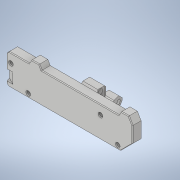
# Autodesk Inventor part: MINI-y-plate-rear
Saved by Autodesk Inventor 2021 (Build 250183000, 183)
## iProperties
Company: Prusa Development a.s.
RuleStatus: InUse
Created: 2019-07-31
Material: Všeobecné
Document SubType Name: Modeling
Density: 1 g/cm^3
Appearance: Výchozí
Project: ORIGINAL PRUSA MINI
Authority: Ing. Robert Turinský
Author: Ing. Robert Turinský
Title: MINI-y-plate-rear
Revision Number: R4
Autodesk Inventor part; units mm, degrees
(part 1 of 2)
ref_plane "XY Plane" through (0, 0, 0) normal (0, 0, 1) x (1, 0, 0)
sketch "Náčrt1" plane through (0, 0, 0) normal (0, 0, 1) x (1, 0, 0)
  line L0 (0, -49.6) -> (0, 14.1) projected
  line L1 (-71.6, 0) -> (163.6, 0) projected
  arc A0 (0.375, -4.0577) -> (-0.375, -4.0577) centre (0, 0) ccw
  arc A1 (120.375, -4.0577) -> (119.625, -4.0577) centre (120, 0) ccw
  line L2 (5, 5) -> (-5, 5)
  line L3 (-5, 5) -> (-8.1754, -0.5)
  line L4 (-8.1754, -0.5) -> (-35.5, -0.5)
  line L5 (-35.5, -0.5) -> (-38, -3)
  line L6 (-38, -3) -> (-38, -38)
  line L7 (-38, -38) -> (-35.5, -40.5)
  line L8 (-35.5, -40.5) -> (114, -40.5)
  line L9 (114, -40.5) -> (130, -24.5)
  line L10 (130, -24.5) -> (130, -3.6603)
  line L11 (130, -3.6603) -> (125, 5)
  line L12 (125, 5) -> (115, 5)
  line L13 (115, 5) -> (111.8246, -0.5)
  line L14 (111.8246, -0.5) -> (8.1754, -0.5)
  line L15 (8.1754, -0.5) -> (5, 5)
  circle A2 centre (87.45, -12.35) radius 2.65
  circle A3 centre (110.7, -35.6) radius 2.65
  circle A4 centre (-32.55, -12.35) radius 2.65
  circle A5 centre (-9.3, -35.6) radius 2.65
  line L16 (119.625, -4.0577) -> (119.625, -12)
  line L17 (119.625, -12) -> (120.375, -12)
  line L18 (120.375, -12) -> (120.375, -4.0577)
  line L19 (-0.375, -4.0577) -> (-0.375, -12)
  line L20 (-0.375, -12) -> (0.375, -12)
  line L21 (0.375, -12) -> (0.375, -4.0577)
  point P0 (120, 5)
  point P1 (0, 5)
  dimension "d0" = 8.15
  dimension "d1" = 120
  dimension "d2" = 0.5
  dimension "d3" = 5.5
  dimension "d4" = 10
  dimension "d5" = 60
  dimension "d6" = 2.5
  dimension "d7" = 2.5
  dimension "d8" = 38
  dimension "d9" = 40.5
  dimension "d10" = 168
  dimension "d11" = 16
  dimension "d12" = 5.3
  dimension "d13" = 5.45
  dimension "d14" = 28.15
  dimension "d15" = 23.25
  dimension "d16" = 23.25
  dimension "d17" = 23.25
  dimension "d18" = 120
  dimension "d25" = 0.75
  dimension "d26" = 12
  constraints: 40 end point, 7 equal length, 6 centre point, 6 parallel, 5 point on line, 4 equal radius, 4 point on circle, 3 perpendicular, 2 horizontal alignment, 2 midpoint, 2 vertical, 2 vertical alignment, 1 coincident, 1 collinear, 1 horizontal
  measures "d0" diameter of A0
  measures "d1" distance of A0.centre A1.centre
  measures "d2" distance between parallel lines of L1 L4
  measures "d3" distance between parallel lines of L4 L2
  measures "d4" distance of L2.start L2.end
  measures "d5" angle of L2 L3
  measures "d6" horizontal distance of L4.end L5.end
  measures "d7" horizontal distance of L4.end L5.end
  measures "d8" distance between parallel lines of L6 L0
  measures "d9" distance between parallel lines of L8 L1
  measures "d10" distance between parallel lines of L6 L10
  measures "d11" horizontal distance of L8.end L9.end
  measures "d12" diameter of A2
  measures "d13" distance from line of L6 A4.centre
  measures "d14" distance from line of L8 A4.centre
  measures "d15" horizontal distance of A5.centre A4.centre
  measures "d16" horizontal distance of A4.centre A5.centre
  measures "d17" horizontal distance of A2.centre A3.centre
  measures "d18" distance of A4.centre A2.centre
  measures "d25" distance between parallel lines of L16 L18
  measures "d26" distance between parallel lines of L17 L1
extrude "Vysunutí1" add sketch "Náčrt1" along normal blind 11.95 contours L8 L7 L6 L5 L4 L3 L1 A0 L19 L20 L0 | L0 L20 L21 A0 L1 L15 L14 L13 A1 L16 L17 L18 L11 L10 L9 L8 | A0 L1 L3 L2 L0 | L0 L2 L15 L1 A0 | L1 A1 L13 L12 L11
extrude "Vysunutí2" [suppressed]
sketch "Náčrt2" plane through (0, 0, 11.95) normal (0, 0, 1) x (1, 0, 0)
  arc A0 (120.375, -4.0577) -> (119.625, -4.0577) centre (120, 0) ccw projected
  arc A1 (0.375, -4.0577) -> (-0.375, -4.0577) centre (0, 0) ccw projected
  circle A2 centre (-9.3, -35.6) radius 2.65 projected
  circle A3 centre (-32.55, -12.35) radius 2.65 projected
  circle A4 centre (110.7, -35.6) radius 2.65 projected
  circle A5 centre (87.45, -12.35) radius 2.65 projected
  line L0 (5, 5) -> (-5, 5) projected
  line L1 (-5, 5) -> (-8.1754, -0.5) projected
  line L2 (-8.1754, -0.5) -> (-35.5, -0.5) projected
  line L3 (-35.5, -0.5) -> (-38, -3) projected
  line L4 (-38, -3) -> (-38, -38) projected
  line L5 (-38, -38) -> (-35.5, -40.5) projected
  line L6 (-35.5, -40.5) -> (114, -40.5) projected
  line L7 (114, -40.5) -> (130, -24.5) projected
  line L8 (130, -24.5) -> (130, -3.6603) projected
  line L9 (130, -3.6603) -> (125, 5) projected
  line L10 (125, 5) -> (115, 5) projected
  line L11 (115, 5) -> (111.8246, -0.5) projected
  line L12 (111.8246, -0.5) -> (8.1754, -0.5) projected
  line L13 (8.1754, -0.5) -> (5, 5) projected
  line L14 (120.375, -4.0577) -> (120.375, -12) projected
  line L15 (120.375, -12) -> (119.625, -12) projected
  line L16 (119.625, -12) -> (119.625, -4.0577) projected
  line L17 (0.375, -4.0577) -> (0.375, -12) projected
  line L18 (0.375, -12) -> (-0.375, -12) projected
  line L19 (-0.375, -12) -> (-0.375, -4.0577) projected
extrude "Vysunutí3" add sketch "Náčrt2" against normal blind 2 contours L14 L15 L16 A0 | L17 L18 L19 A1
ref_plane "Pracovní rovina1" through (50, 0, 0) normal (1, 0, 0) x (0, 1, 0)
sketch "Náčrt3" plane through (50, 0, 0) normal (1, 0, 0) x (0, 1, 0)
  line L0 (-0.5, 0) -> (-0.5, 11.95) projected
  line L1 (-48.9, 0) -> (9.9, 0) projected
  line L2 (0, -53.99) -> (0, 22.94) projected
  circle A0 centre (-18, -21) radius 11.25
  line L3 (-0.5, 0) -> (1.5, -2)
  line L4 (1.5, -2) -> (1.5, -11)
  line L5 (1.5, -11) -> (-0.5, -13)
  line L6 (-0.5, -13) -> (-10.0904, -13)
  line L7 (-26.5, -28.3697) -> (-26.5, -37)
  line L8 (-26.5, -37) -> (-32.5, -43)
  line L9 (-32.5, -43) -> (-36, -43)
  line L10 (-36, -43) -> (-39, -40)
  line L11 (-39, -40) -> (-40.5, -27)
  line L12 (-40.5, -27) -> (-40.5, 0)
  line L13 (-0.5, 0) -> (-0.5, 11.95) projected
  line L14 (-40.5, 0) -> (-0.5, 0)
  line L15 (-40.5, 0) -> (-40.5, 11.95) projected
  circle A1 centre (-2.5, -5.5) radius 1.7
  circle A2 centre (-33.5, -5.5) radius 1.7
  circle A3 centre (-33.5, -36.5) radius 1.7
  point P0 (0, 0)
  dimension "d28" = 22.5
  dimension "d29" = 21
  dimension "d30" = 18
  dimension "d31" = 8
  dimension "d32" = 19.5
  dimension "d33" = 45
  dimension "d34" = 8.5
  dimension "d35" = 6
  dimension "d36" = 22
  dimension "d37" = 3
  dimension "d38" = 13
  dimension "d39" = 1.5
  dimension "d40" = 3.4
  dimension "d41" = 31
  dimension "d42" = 31
  dimension "d43" = 15.5
  dimension "d44" = 15.5
  constraints: 22 end point, 5 perpendicular, 4 centre point, 3 vertical, 2 equal radius, 2 horizontal, 2 point on circle, 2 point on line, 1 horizontal alignment, 1 vertical alignment
  measures "d28" diameter of A0
  measures "d29" distance from line of L1 A0.centre
  measures "d30" distance from line of L2 A0.centre
  measures "d31" distance from line of A0.centre L6
  measures "d32" distance from line of A0.centre L4
  measures "d33" angle of L1 L3
  measures "d34" distance from line of L7 A0.centre
  measures "d35" horizontal distance of L7.end L8.end
  measures "d36" distance from line of A0.centre L9
  measures "d37" horizontal distance of L9.end L10.end
  measures "d38" vertical distance of L10.end L11.end
  measures "d39" horizontal distance of L10.end L11.end
  measures "d40" diameter of A1
  measures "d41" distance of A2.centre A1.centre
  measures "d42" distance of A3.centre A2.centre
  measures "d43" horizontal distance of A0.centre A2.centre
  measures "d44" horizontal distance of A0.centre A2.centre
extrude "Vysunutí4" add sketch "Náčrt3" along normal blind 20 contours L1 L3 L2 L5 L6 A0 L7 L8 L9 L10 L11 L12 | L3 L4 L5 L2
sketch "Náčrt4" plane through (0, 0, 0) normal (0, 1, 0) x (-1, 0, 0)
  line L0 (35.5, 0) -> (-50, 0) projected
  line L1 (-50, 0) -> (-50, -27) projected
  line L2 (-50, -27) -> (-70, -27) projected
  line L3 (-70, 0) -> (-70, -27) projected
  line L4 (-70, 0) -> (-114, 0) projected
  line L5 (-114, 0) -> (-114, 11.95) projected
  line L6 (35.5, 11.95) -> (-114, 11.95) projected
  line L7 (35.5, 0) -> (35.5, 11.95) projected
  line L8 (-50, -27) -> (-50, -40) projected
  line L9 (-50, -40) -> (-70, -40) projected
  line L10 (-70, -27) -> (-70, -40) projected
  line L11 (-50, -27) -> (-70, -27) projected
  line L12 (-50, -40) -> (-50, -43) projected
  line L13 (-50, -43) -> (-70, -43) projected
  line L14 (-70, -40) -> (-70, -43) projected
  line L15 (-50, -40) -> (-70, -40) projected
  line L16 (-61.5, -43) -> (-70, -43)
  line L17 (-70, -43) -> (-70, -11.2776)
  line L18 (-70, -11) -> (-70, -2) projected
  line L19 (-70, -11.2776) -> (-61.5, -43)
  point P0 (0, 0)
  dimension "d47" = 15
  dimension "d48" = 8.5
  constraints: 6 end point, 2 point on line, 1 horizontal
  measures "d47" angle of L14 L19
  measures "d48" horizontal distance of L17.end L16.start
extrude "Vysunutí5" cut sketch "Náčrt4" along normal through all both and the other way through all contours L19 L9 L10 L2 | L2 L3 L19 | L19 L13 L14 L9
sketch "Náčrt5" plane through (70, 0, 0) normal (1, 0, 0) x (0, 0, -1)
  point P0 (0, 0)
  point P1 (5.5, -2.5)
  point P2 (5.5, -33.5)
  point P3 (36.5, -33.5)
hole "Díra1" at (70, -2.5, -5.5) at (70, -33.5, -5.5) at (70, -33.5, -36.5) direction (-1, 0, 0) diameter 3.4 end through all counterbore diameter 6 counterbore depth 11
ref_plane "Pracovní rovina2" through (0, -23.975, 0) normal (0, 1, 0) x (-1, 0, 0)
sketch "Náčrt6" plane through (0, -23.975, 0) normal (0, 1, 0) x (-1, 0, 0)
  line L0 (-111.8246, 0) -> (-70, 0) projected
  line L1 (-115, 0) -> (-111.8246, 0) projected
  line L2 (-125, 0) -> (-115, 0) projected
  line L3 (-130, 0) -> (-125, 0) projected
  line L4 (-114, 0) -> (-130, 0) projected
  line L5 (-70, 0) -> (-114, 0) projected
  line L6 (-120.375, 0) -> (-119.625, 0) projected
  line L7 (-119.625, 0) -> (-120.375, 0) projected
  line L8 (-108.05, 0) -> (-113.35, 0) projected
  line L9 (-84.8, 0) -> (-90.1, 0) projected
  line L10 (-70, -8.5) -> (-70, -2.5) projected
  line L11 (-70, -8.5) -> (-70, -2.5) projected
  line L12 (-70, -11.2776) -> (-70, -11) projected
  line L13 (-70, -11) -> (-70, -2) projected
  line L14 (-70, -2) -> (-70, 0) projected
  line L15 (-70, 0) -> (-70, -11.2776) projected
  line L16 (-70, -11.2776) -> (-70, -11.2776) projected
  line L17 (-50, -34.8) -> (-50, -38.2) projected
  line L18 (-50, -3.8) -> (-50, -7.2) projected
  line L19 (-50, -3.8) -> (-50, -7.2) projected
  line L20 (-50, -2) -> (-50, 0) projected
  line L21 (-50, -11) -> (-50, -2) projected
  line L22 (-50, -13) -> (-50, -11) projected
  line L23 (-50, -28.3697) -> (-50, -13) projected
  line L24 (-50, -37) -> (-50, -28.3697) projected
  line L25 (-50, -43) -> (-50, -37) projected
  line L26 (-50, -40) -> (-50, -43) projected
  line L27 (-50, -27) -> (-50, -40) projected
  line L28 (-50, 0) -> (-50, -27) projected
  line L29 (-0.375, 0) -> (0.375, 0) projected
  line L30 (0.375, 0) -> (-0.375, 0) projected
  line L31 (11.95, 0) -> (6.65, 0) projected
  line L32 (35.2, 0) -> (29.9, 0) projected
  line L33 (35.5, 0) -> (-50, 0) projected
  line L34 (38, 0) -> (35.5, 0) projected
  line L35 (35.5, 0) -> (38, 0) projected
  line L36 (8.1754, 0) -> (35.5, 0) projected
  line L37 (5, 0) -> (8.1754, 0) projected
  line L38 (-5, 0) -> (5, 0) projected
  line L39 (-8.1754, 0) -> (-5, 0) projected
  line L40 (-50, 0) -> (-8.1754, 0) projected
  line L41 (-70, 0) -> (-50, 0) projected
  line L42 (-70, 0) -> (-93, 0)
  line L43 (-93, 0) -> (-93, -11)
  line L44 (-93, -11) -> (-70, -11)
  line L45 (-70, -11) -> (-70, 0)
  line L46 (11.95, 0) -> (6.65, 0) projected
  line L47 (15, 0) -> (-9, 0)
  line L48 (-9, 0) -> (-9, -11)
  line L49 (-9, -11) -> (15, -11)
  line L50 (15, -11) -> (15, 0)
  line L51 (0, -51.6) -> (0, 8.6) projected
  line L52 (-9, -11) -> (-9, -17)
  line L53 (-9, -17) -> (15, -11)
  point P0 (0, 0)
  dimension "d59" = 11
  dimension "d60" = 41
  dimension "d61" = 93
  dimension "d62" = 15
  dimension "d235" = 17
  constraints: 20 end point, 4 parallel, 2 horizontal, 2 perpendicular, 1 collinear, 1 point on line, 1 vertical
  measures "d59" distance between parallel lines of L0 L44
  measures "d60" distance between parallel lines of L21 L48
  measures "d61" distance between parallel lines of L43 L51
  measures "d62" distance between parallel lines of L50 L51
  measures "d235" distance from line of L33 L52.end
extrude "Vysunutí6" add sketch "Náčrt6" along normal mid plane 7.5
chamfer "Zkosení1" distance 1 angle 45 10 edges at (81.5, -20.225, -11) (81.5, -27.725, -11) (93, -20.225, -5.5) (93, -23.975, -11) (93, -27.725, -5.5) (-15, -20.225, -5.5) (-15, -23.975, -11) (-15, -27.725, -5.5) (-3, -20.225, -14) (-3, -27.725, -14)
chamfer "Zkosení2" distance 2 angle 45 2 edges at (70, -10.3625, 0) (70, -34.1125, 0)
ref_plane "Pracovní rovina3" through (0, 0, 10.95) normal (0, 0, 1) x (1, 0, 0)
ref_plane "Pracovní rovina6" through (9.2425, -26.725, -16.0299) normal (-0.2425356, 0, -0.9701425) x (-0.9701425, 0, 0.2425356)
sketch "Náčrt8" plane through (0, 0, 10.95) normal (0, 0, 1) x (1, 0, 0)
  circle A0 centre (-9.3, -35.6) radius 2.65 projected
  circle A1 centre (-32.55, -12.35) radius 2.65 projected
  circle A2 centre (110.7, -35.6) radius 2.65 projected
  circle A3 centre (87.45, -12.35) radius 2.65 projected
  line L0 (5, 5) -> (-5, 5) projected
  line L1 (-5, 5) -> (-8.1754, -0.5) projected
  line L2 (-8.1754, -0.5) -> (-35.5, -0.5) projected
  line L3 (-35.5, -0.5) -> (-38, -3) projected
  line L4 (-38, -3) -> (-38, -38) projected
  line L5 (-38, -38) -> (-35.5, -40.5) projected
  line L6 (-35.5, -40.5) -> (114, -40.5) projected
  line L7 (114, -40.5) -> (130, -24.5) projected
  line L8 (130, -24.5) -> (130, -3.6603) projected
  line L9 (130, -3.6603) -> (125, 5) projected
  line L10 (125, 5) -> (115, 5) projected
  line L11 (115, 5) -> (111.8246, -0.5) projected
  line L12 (111.8246, -0.5) -> (8.1754, -0.5) projected
  line L13 (8.1754, -0.5) -> (5, 5) projected
  arc A4 (120.375, -4.0577) -> (119.625, -4.0577) centre (120, 0) ccw projected
  line L14 (120.375, -12) -> (120.375, -4.0577) projected
  line L15 (119.625, -12) -> (120.375, -12) projected
  line L16 (119.625, -4.0577) -> (119.625, -12) projected
  arc A5 (0.375, -4.0577) -> (-0.375, -4.0577) centre (0, 0) ccw projected
  line L17 (0.375, -12) -> (0.375, -4.0577) projected
  line L18 (-0.375, -12) -> (0.375, -12) projected
  line L19 (-0.375, -4.0577) -> (-0.375, -12) projected
  line L20 (114.8921, -2.14) -> (5.1079, -2.14)
  line L21 (5.1079, -2.14) -> (5.1079, -2.24)
  line L22 (5.1079, -2.24) -> (114.8921, -2.24)
  line L23 (114.8921, -2.24) -> (114.8921, -2.14)
  line L24 (117.1145, -3.88) -> (2.8855, -3.88)
  line L25 (2.8855, -3.88) -> (2.8855, -3.98)
  line L26 (2.8855, -3.98) -> (117.1145, -3.98)
  line L27 (117.1145, -3.98) -> (117.1145, -3.88)
  line L28 (117.985, -5.62) -> (2.015, -5.62)
  line L29 (2.015, -5.62) -> (2.015, -5.72)
  line L30 (2.015, -5.72) -> (117.985, -5.72)
  line L31 (117.985, -5.72) -> (117.985, -5.62)
  line L32 (70, -20.225) -> (92, -20.225) projected
  line L33 (92, -27.725) -> (70, -27.725) projected
  line L34 (128.36, -21.075) -> (-36.36, -21.075)
  line L35 (-36.36, -21.075) -> (-36.36, -21.175)
  line L36 (-36.36, -21.175) -> (128.36, -21.175)
  line L37 (128.36, -21.175) -> (128.36, -21.075)
  line L38 (125.985, -26.775) -> (-36.36, -26.775)
  line L39 (-36.36, -26.775) -> (-36.36, -26.875)
  line L40 (-36.36, -26.875) -> (125.985, -26.875)
  line L41 (125.985, -26.875) -> (125.985, -26.775)
  line L42 (128.36, -22.965) -> (-36.36, -22.965)
  line L43 (-36.36, -22.965) -> (-36.36, -23.065)
  line L44 (-36.36, -23.065) -> (128.36, -23.065)
  line L45 (128.36, -23.065) -> (128.36, -22.965)
  line L46 (127.875, -24.885) -> (-36.36, -24.885)
  line L47 (-36.36, -24.885) -> (-36.36, -24.985)
  line L48 (-36.36, -24.985) -> (127.875, -24.985)
  line L49 (127.875, -24.985) -> (127.875, -24.885)
  line L50 (93, -21.225) -> (93, -26.725) projected
  line L51 (-14, -27.725) -> (9, -27.725) projected
  line L52 (9, -27.725) -> (9, -20.225) projected
  line L53 (9, -20.225) -> (-14, -20.225) projected
  line L54 (-15, -21.225) -> (-14, -20.225) projected
  line L55 (-15, -21.225) -> (-15, -26.725) projected
  line L56 (-14, -27.725) -> (-15, -26.725) projected
  arc A6 (0.375, -4.0577) -> (-0.375, -4.0577) centre (0, 0) ccw projected
  line L57 (-0.375, -4.0577) -> (-0.375, -12) projected
  line L58 (-0.375, -12) -> (0.375, -12) projected
  line L59 (0.375, -12) -> (0.375, -4.0577) projected
  circle A7 centre (-9.3, -35.6) radius 2.65 projected
  circle A8 centre (-32.55, -12.35) radius 2.65 projected
  line L60 (50, -0.5) -> (50, -40.5) projected
  line L61 (-35.5, -40.5) -> (50, -40.5) projected
  line L62 (-38, -38) -> (-35.5, -40.5) projected
  line L63 (-38, -3) -> (-38, -38) projected
  line L64 (-35.5, -0.5) -> (-38, -3) projected
  line L65 (-8.1754, -0.5) -> (-35.5, -0.5) projected
  line L66 (-5, 5) -> (-8.1754, -0.5) projected
  line L67 (5, 5) -> (-5, 5) projected
  line L68 (8.1754, -0.5) -> (5, 5) projected
  line L69 (50, -0.5) -> (8.1754, -0.5) projected
  line L70 (10, -20.225) -> (10, -27.725) projected
  line L71 (-15, -26.725) -> (-15, -21.225) projected
  line L72 (91.36, -21.075) -> (51.64, -21.075)
  line L73 (51.64, -21.075) -> (51.64, -21.175)
  line L74 (51.64, -21.175) -> (91.36, -21.175)
  line L75 (91.36, -21.175) -> (91.36, -21.075)
  line L76 (51.64, -22.965) -> (91.36, -22.965)
  line L77 (91.36, -22.965) -> (91.36, -23.065)
  line L78 (91.36, -23.065) -> (51.64, -23.065)
  line L79 (51.64, -23.065) -> (51.64, -22.965)
  line L80 (91.36, -24.885) -> (51.64, -24.885)
  line L81 (51.64, -24.885) -> (51.64, -24.985)
  line L82 (51.64, -24.985) -> (91.36, -24.985)
  line L83 (91.36, -24.985) -> (91.36, -24.885)
  line L84 (51.64, -26.775) -> (91.36, -26.775)
  line L85 (91.36, -26.775) -> (91.36, -26.875)
  line L86 (91.36, -26.875) -> (51.64, -26.875)
  line L87 (51.64, -26.875) -> (51.64, -26.775)
  line L88 (7.36, -21.075) -> (-13.36, -21.075)
  line L89 (-13.36, -21.075) -> (-13.36, -21.175)
  line L90 (-13.36, -21.175) -> (7.36, -21.175)
  line L91 (7.36, -21.175) -> (7.36, -21.075)
  line L92 (-13.36, -22.965) -> (7.36, -22.965)
  line L93 (7.36, -22.965) -> (7.36, -23.065)
  line L94 (7.36, -23.065) -> (-13.36, -23.065)
  line L95 (-13.36, -23.065) -> (-13.36, -22.965)
  line L96 (7.36, -24.885) -> (-13.36, -24.885)
  line L97 (-13.36, -24.885) -> (-13.36, -24.985)
  line L98 (-13.36, -24.985) -> (7.36, -24.985)
  line L99 (7.36, -24.985) -> (7.36, -24.885)
  line L100 (-13.36, -26.775) -> (7.36, -26.775)
  line L101 (7.36, -26.775) -> (7.36, -26.875)
  line L102 (7.36, -26.875) -> (-13.36, -26.875)
  line L103 (-13.36, -26.875) -> (-13.36, -26.775)
  line L104 (-36.36, -29.7879) -> (122.9721, -29.7879)
  line L105 (122.9721, -29.7879) -> (122.9721, -29.8879)
  line L106 (122.9721, -29.8879) -> (-36.36, -29.8879)
  line L107 (-36.36, -29.8879) -> (-36.36, -29.7879)
  line L108 (114, -40.5) -> (130, -24.5) projected
  line L109 (105.7, -32.8007) -> (-4.3, -32.8007)
  line L110 (-4.3, -32.8007) -> (-4.3, -32.9007)
  line L111 (-4.3, -32.9007) -> (105.7, -32.9007)
  line L112 (105.7, -32.9007) -> (105.7, -32.8007)
  line L113 (-14.3, -32.8007) -> (-36.36, -32.8007)
  line L114 (-36.36, -32.8007) -> (-36.36, -32.9007)
  line L115 (-36.36, -32.9007) -> (-14.3, -32.9007)
  line L116 (-14.3, -32.9007) -> (-14.3, -32.8007)
  line L117 (-36.36, -35.7136) -> (-36.36, -35.8136)
  line L118 (-14.3, -35.7136) -> (-36.36, -35.7136)
  line L119 (-14.3, -35.8136) -> (-14.3, -35.7136)
  line L120 (-36.36, -35.8136) -> (-14.3, -35.8136)
  line L121 (-4.3, -35.8136) -> (105.7, -35.8136)
  line L122 (105.7, -35.7136) -> (-4.3, -35.7136)
  line L123 (105.7, -35.8136) -> (105.7, -35.7136)
  line L124 (-4.3, -35.7136) -> (-4.3, -35.8136)
  line L125 (-36.36, -38.6265) -> (-36.36, -38.7265)
  line L126 (-14.3, -38.6265) -> (-36.36, -38.6265)
  line L127 (-14.3, -38.7265) -> (-14.3, -38.6265)
  line L128 (-36.36, -38.7265) -> (-14.3, -38.7265)
  line L129 (-4.3, -38.7265) -> (105.7, -38.7265)
  line L130 (105.7, -38.6265) -> (-4.3, -38.6265)
  line L131 (105.7, -38.7265) -> (105.7, -38.6265)
  line L132 (-4.3, -38.6265) -> (-4.3, -38.7265)
  line L133 (-35.6335, -38.6265) -> (-14.3, -38.6265)
  line L134 (-14.3, -38.6265) -> (-14.3, -38.7265)
  line L135 (-14.3, -38.7265) -> (-35.6335, -38.7265)
  line L136 (-35.6335, -38.7265) -> (-35.6335, -38.6265)
  line L137 (128.36, -18.0621) -> (-36.36, -18.0621)
  line L138 (-36.36, -18.0621) -> (-36.36, -18.1621)
  line L139 (-36.36, -18.1621) -> (128.36, -18.1621)
  line L140 (128.36, -18.1621) -> (128.36, -18.0621)
  line L141 (-27.55, -15.0493) -> (82.45, -15.0493)
  line L142 (82.45, -15.0493) -> (82.45, -15.1493)
  line L143 (82.45, -15.1493) -> (-27.55, -15.1493)
  line L144 (-27.55, -15.1493) -> (-27.55, -15.0493)
  line L145 (92.45, -15.0493) -> (128.36, -15.0493)
  line L146 (128.36, -15.0493) -> (128.36, -15.1493)
  line L147 (128.36, -15.1493) -> (92.45, -15.1493)
  line L148 (92.45, -15.1493) -> (92.45, -15.0493)
  line L149 (128.36, -12.0364) -> (122.015, -12.0364)
  line L150 (122.015, -12.0364) -> (122.015, -12.1364)
  line L151 (122.015, -12.1364) -> (128.36, -12.1364)
  line L152 (128.36, -12.1364) -> (128.36, -12.0364)
  line L153 (117.985, -12.0364) -> (92.45, -12.0364)
  line L154 (92.45, -12.0364) -> (92.45, -12.1364)
  line L155 (92.45, -12.1364) -> (117.985, -12.1364)
  line L156 (117.985, -12.1364) -> (117.985, -12.0364)
  line L157 (82.45, -12.0364) -> (2.015, -12.0364)
  line L158 (2.015, -12.0364) -> (2.015, -12.1364)
  line L159 (2.015, -12.1364) -> (82.45, -12.1364)
  line L160 (82.45, -12.1364) -> (82.45, -12.0364)
  line L161 (-2.015, -12.0364) -> (-27.55, -12.0364)
  line L162 (-27.55, -12.0364) -> (-27.55, -12.1364)
  line L163 (-27.55, -12.1364) -> (-2.015, -12.1364)
  line L164 (-2.015, -12.1364) -> (-2.015, -12.0364)
  line L165 (-27.55, -9.1235) -> (-27.55, -9.2235)
  line L166 (-27.55, -9.2235) -> (-2.015, -9.2235)
  line L167 (-2.015, -9.1235) -> (-27.55, -9.1235)
  line L168 (-2.015, -9.2235) -> (-2.015, -9.1235)
  line L169 (2.015, -9.2235) -> (82.45, -9.2235)
  line L170 (82.45, -9.1235) -> (2.015, -9.1235)
  line L171 (82.45, -9.2235) -> (82.45, -9.1235)
  line L172 (2.015, -9.1235) -> (2.015, -9.2235)
  line L173 (92.45, -9.1235) -> (92.45, -9.2235)
  line L174 (117.985, -9.1235) -> (92.45, -9.1235)
  line L175 (92.45, -9.2235) -> (117.985, -9.2235)
  line L176 (117.985, -9.2235) -> (117.985, -9.1235)
  line L177 (122.015, -9.1235) -> (122.015, -9.2235)
  line L178 (128.36, -9.1235) -> (122.015, -9.1235)
  line L179 (122.015, -9.2235) -> (128.36, -9.2235)
  line L180 (128.36, -9.2235) -> (128.36, -9.1235)
  line L181 (-2.015, -6.3107) -> (-2.015, -6.2107)
  line L182 (-27.55, -6.2107) -> (-27.55, -6.3107)
  line L183 (-2.015, -6.2107) -> (-27.55, -6.2107)
  line L184 (-27.55, -6.3107) -> (-2.015, -6.3107)
  line L185 (-27.55, -6.2107) -> (-36.36, -6.2107)
  line L186 (-36.36, -6.2107) -> (-36.36, -6.3107)
  line L187 (-36.36, -6.3107) -> (-27.55, -6.3107)
  line L188 (-27.55, -6.3107) -> (-27.55, -6.2107)
  line L189 (-36.36, -3.1978) -> (-7.5258, -3.1978)
  line L190 (-7.5258, -3.1978) -> (-7.5258, -3.2978)
  line L191 (-7.5258, -3.2978) -> (-36.36, -3.2978)
  line L192 (-36.36, -3.2978) -> (-36.36, -3.1978)
  line L193 (122.015, -6.2107) -> (128.36, -6.2107)
  line L194 (128.36, -6.2107) -> (128.36, -6.3107)
  line L195 (128.36, -6.3107) -> (122.015, -6.3107)
  line L196 (122.015, -6.3107) -> (122.015, -6.2107)
  line L197 (2.015, -6.2107) -> (117.985, -6.2107)
  line L198 (117.985, -6.2107) -> (117.985, -6.3107)
  line L199 (117.985, -6.3107) -> (2.015, -6.3107)
  line L200 (2.015, -6.3107) -> (2.015, -6.2107)
  line L201 (7.5258, -3.1978) -> (112.4742, -3.1978)
  line L202 (112.4742, -3.1978) -> (112.4742, -3.2978)
  line L203 (112.4742, -3.2978) -> (7.5258, -3.2978)
  line L204 (7.5258, -3.2978) -> (7.5258, -3.1978)
  line L205 (124.1658, -3.1978) -> (128.093, -3.1978)
  line L206 (128.093, -3.1978) -> (128.093, -3.2978)
  line L207 (128.093, -3.2978) -> (124.1658, -3.2978)
  line L208 (124.1658, -3.2978) -> (124.1658, -3.1978)
  circle A9 centre (87.45, -12.35) radius 3.5
  circle A10 centre (87.45, -12.35) radius 3.6
  circle A11 centre (110.7, -35.6) radius 3.5
  circle A12 centre (110.7, -35.6) radius 3.6
  circle A13 centre (-9.3, -35.6) radius 3.5
  circle A14 centre (-9.3, -35.6) radius 3.6
  circle A15 centre (-32.55, -12.35) radius 3.5
  circle A16 centre (-32.55, -12.35) radius 3.6
  point P0 (116.5321, -2.14)
  point P1 (3.4679, -2.14)
  point P2 (118.7545, -3.88)
  point P3 (1.2455, -3.88)
  point P4 (127.625, -26.875)
  point P5 (129.515, -24.985)
  point P6 (124.6121, -29.8879)
  point P7 (-37.2735, -38.7265)
  point P8 (-2.5258, -3.1978)
  point P9 (2.5258, -3.1978)
  point P10 (117.4742, -3.1978)
  point P11 (129.733, -3.1978)
  point P12 (122.5258, -3.1978)
  dimension "d83" = 0.1
  dimension "d84" = 1.64
  dimension "d86" = 1.64
  dimension "d87" = 1.64
  dimension "d89" = 1.64
  dimension "d90" = 1.64
  dimension "d91" = 1.64
  dimension "d92" = 1.64
  dimension "d93" = 1.64
  dimension "d94" = 1.64
  dimension "d97" = 0.85
  dimension "d98" = 0.85
  dimension "d99" = 1.64
  dimension "d100" = 1.64
  dimension "d101" = 1.64
  dimension "d102" = 1.79
  dimension "d104" = 1.79
  dimension "d105" = 1.64
  dimension "d106" = 1.64
  dimension "d107" = 1.64
  dimension "d108" = 1.64
  dimension "d109" = 1.64
  dimension "d112" = 2.9129
  dimension "d113" = 1.64
  dimension "d114" = 2.9129
  dimension "d115" = 5
  dimension "d116" = 5
  dimension "d117" = 5
  dimension "d120" = 2.9129
  dimension "d125" = 1.64
  dimension "d126" = 2.9129
  dimension "d127" = 5
  dimension "d128" = 5
  dimension "d129" = 5
  dimension "d130" = 2.9129
  dimension "d131" = 2.9129
  dimension "d132" = 1.64
  dimension "d133" = 1.64
  dimension "d134" = 1.64
  dimension "d135" = 1.64
  dimension "d138" = 2.9129
  dimension "d145" = 2.9129
  dimension "d150" = 2.9129
  dimension "d151" = 5
  dimension "d152" = 5
  dimension "d153" = 5
  dimension "d154" = 1.64
  dimension "d155" = 1.64
  dimension "d156" = 0.85
  dimension "d157" = 0.1
  constraints: 328 end point, 64 parallel, 55 point on line, 34 collinear, 32 horizontal, 32 perpendicular, 12 equal length, 8 centre point, 8 point on circle, 6 equal radius, 3 vertical, 1 vertical alignment, 72 other
  measures "d83" distance between parallel lines of L22 L20
  measures "d84" distance between parallel lines of L20 L12
  measures "d86" distance of L20.start point (116.532, -2.14)
  measures "d87" distance of point (3.468, -2.14) L20.end
  measures "d89" distance between parallel lines of L24 L22
  measures "d90" distance from line of L27 point (118.755, -3.88)
  measures "d91" distance from line of L25 point (1.245, -3.88)
  measures "d92" distance between parallel lines of L28 L26
  measures "d93" distance between parallel lines of L16 L31
  measures "d94" distance between parallel lines of L29 L17
  measures "d97" distance between parallel lines of L32 L34
  measures "d98" distance between parallel lines of L33 L40
  measures "d99" distance between parallel lines of L8 L37
  measures "d100" distance from line of point (127.625, -26.875) L41
  measures "d101" distance between parallel lines of L4 L39
  measures "d102" distance between parallel lines of L42 L36
  measures "d104" distance between parallel lines of L38 L48
  measures "d105" distance from line of L49 point (129.515, -24.985)
  measures "d106" distance between parallel lines of L75 L50
  measures "d107" distance between parallel lines of L60 L73
  measures "d108" distance between parallel lines of L91 L52
  measures "d109" distance between parallel lines of L89 L71
  measures "d112" distance between parallel lines of L104 L40
  measures "d113" distance from line of L105 point (124.612, -29.888)
  measures "d114" distance between parallel lines of L106 L109
  measures "d115" distance from line of A7.centre L116
  measures "d116" distance from line of A0.centre L110
  measures "d117" distance from line of L112 A2.centre
  measures "d120" distance of L113.end L117.start
  measures "d125" distance from line of L136 point (-37.274, -38.726)
  measures "d126" distance between parallel lines of L34 L139
  measures "d127" distance from line of A1.centre L144
  measures "d128" distance from line of A3.centre L142
  measures "d129" distance from line of A3.centre L148
  measures "d130" distance between parallel lines of L137 L147
  measures "d131" distance between parallel lines of L145 L151
  measures "d132" distance between parallel lines of L14 L150
  measures "d133" distance between parallel lines of L16 L156
  measures "d134" distance between parallel lines of L17 L158
  measures "d135" distance between parallel lines of L19 L164
  measures "d138" distance of L162.end L165.end
  measures "d145" distance of L165.end L182.end
  measures "d150" distance between parallel lines of L185 L191
  measures "d151" distance from line of L190 point (-2.526, -3.198)
  measures "d152" distance from line of point (2.526, -3.198) L204
  measures "d153" distance from line of L202 point (117.474, -3.198)
  measures "d154" distance from line of point (122.526, -3.198) L208
  measures "d155" distance from line of point (129.733, -3.198) L206
  measures "d156" radial gap between concentric circles of A3 A9
  measures "d157" radial gap between concentric circles of A9 A10
extrude "Vysunutí8" cut sketch "Náčrt8" against normal blind 9.95 contours L111 L110 L109 L60 | L60 L109 L112 L111 | L170 L171 L169 L60 | L60 L169 L172 L170 | L60 L38 L87 L40 | L40 L70 L38 L60 | L40 L52 L38 L70 | L87 L38 L85 L40 | L40 L101 L38 L52 | L85 L38 L41 L40 | L60 L46 L81 L48 | L48 L70 L46 L60 | L40 L103 L38 L101 | L48 L52 L46 L70 | L81 L46 L83 L48 | L40 L56 L38 L103 | L48 L99 L46 L52 | L83 L46 L50 L48 | L60 L42 L79 L44 | L44 L70 L42 L60 | L40 L39 L38 L56 | L48 L97 L46 L99 | L44 L52 L42 L70 | L50 L46 L49 L48 | L79 L42 L77 L44 | L60 L36 L70 L34 | L34 L73 L36 L60 | L48 L55 L46 L97 | L44 L93 L42 L52 | L77 L42 L50 L44 | L34 L75 L36 L73 | L70 L36 L52 L34 | L48 L47 L46 L55 | L44 L95 L42 L93 | L50 L42 L45 L44 | L34 L37 L36 L75 | L52 L36 L91 L34 | L44 L55 L42 L95 | L91 L36 L89 L34 | L44 L43 L42 L55 | L89 L36 L54 L34 | L54 L36 L35 L34 | L116 L115 L114 L113 | L167 L168 L166 L165 | L174 L176 L175 L173 | L178 L180 L179 L177 | A10 | A12 | A14 | A16
extrude "Vysunutí13" cut sketch "Náčrt8" against normal up to surface contours L40 L103 L38 L101 | L48 L97 L46 L99 | L44 L95 L42 L93 | L91 L36 L89 L34 surface through (9.2425, -26.725, -16.0299) normal (-0.2425356, 0, -0.9701425)
extrude "Vysunutí9" cut sketch "Náčrt8" against normal blind 20.95 contours L87 L38 L85 L40 | L81 L46 L83 L48 | L79 L42 L77 L44 | L34 L75 L36 L73
ref_plane "Pracovní rovina4" through (57.65, -2.5, -5.5) normal (1, 0, 0) x (0, 0, -1)
sketch "Náčrt9" plane through (57.65, -2.5, -5.5) normal (1, 0, 0) x (0, 0, -1)
  circle A0 centre (0, 0) radius 1.7 projected
  circle A1 centre (0, -31) radius 1.7 projected
  circle A2 centre (31, -31) radius 1.7 projected
  circle A3 centre (0, 0) radius 2.95
  circle A4 centre (0, -31) radius 2.95
  circle A5 centre (31, -31) radius 2.95
  line L0 (4.7822, 2.95) -> (-2.7822, 2.95)
  line L1 (-4.2, 1.5322) -> (-4.2, -6.95)
  line L2 (-4.2, -6.95) -> (5.37, -6.95)
  line L3 (5.37, -6.95) -> (5.37, 2.3622)
  line L4 (6.95, -25.63) -> (-5.37, -25.63)
  line L5 (-5.37, -25.63) -> (-5.37, -36.37)
  line L6 (-5.37, -36.37) -> (6.95, -36.37)
  line L7 (6.95, -36.37) -> (6.95, -25.63)
  line L8 (35.2, -34.0322) -> (35.2, -29.4678)
  line L9 (35.2, -29.4678) -> (30.9822, -25.25)
  line L10 (37.5, -30) -> (31.5, -24) projected
  line L11 (35.2, -34.0322) -> (33.9241, -35.3082)
  line L12 (34.5, -36.5) -> (37.5, -33.5) projected
  line L13 (-4.2, 1.5322) -> (-2.7822, 2.95)
  line L14 (4.7822, 2.95) -> (5.37, 2.3622)
  line L15 (7.5, 2) -> (5.5, 4) projected
  line L16 (-3.5, 4) -> (-5.5, 2) projected
  line L17 (24.7215, -36.37) -> (6.95, -36.37)
  arc A6 (6.95, -25.63) -> (24.4809, -25.25) centre (15.5, -15.5) ccw
  arc A7 (7.5, -7.5904) -> (22.8697, -24) centre (15.5, -15.5) ccw projected
  line L18 (24.4809, -25.25) -> (30.9822, -25.25)
  line L19 (31.5, -24) -> (22.8697, -24) projected
  line L20 (33.9241, -35.3082) -> (24.7215, -36.37)
  line L21 (-5.5, -38) -> (21.5, -38) projected
  line L22 (21.5, -38) -> (34.5, -36.5) projected
  point P0 (-5.5, 2.5)
  dimension "d160" = 1.25
  dimension "d168" = 1.25
  dimension "d171" = 1.25
  dimension "d172" = 2.42
  dimension "d173" = 2.42
  dimension "d174" = 4
  dimension "d175" = 2.42
  dimension "d176" = 4
  dimension "d177" = 2.42
  dimension "d178" = 1.25
  dimension "d183" = 1.25
  dimension "d184" = 1.25
  dimension "d205" = 1.25
  dimension "d206" = 1.25
  dimension "d207" = 1.25
  constraints: 32 end point, 10 parallel, 4 centre point, 3 horizontal, 2 equal radius, 2 perpendicular, 2 point on circle, 1 concentric, 1 tangent, 1 vertical
  measures "d160" radial gap between concentric circles of A1 A4
  measures "d168" distance between parallel lines of L10 L9
  measures "d171" distance between parallel lines of L12 L11
  measures "d172" distance edge to line of A4 L6
  measures "d173" distance edge to line of A4 L4
  measures "d174" distance edge to line of A4 L7
  measures "d175" distance edge to line of A4 L5
  measures "d176" distance edge to line of A3 L2
  measures "d177" distance edge to line of A3 L3
  measures "d178" distance edge to line of A3 L1
  measures "d183" distance between parallel lines of L13 L16
  measures "d184" distance between parallel lines of L15 L14
  measures "d205" distance between parallel lines of L19 L18
  measures "d206" distance edge to line of A5 L8
  measures "d207" distance between parallel lines of L22 L20
extrude "Vysunutí10" cut sketch "Náčrt9" against normal blind 0.1 contours L0 L14 L3 L2 L1 L13 | L7 L6 L5 L4 | A6 L18 L9 L8 L11 L20 L17 L7
pattern_linear "Obdélníkové pole2" count 5 spacing 1.35 along (-1, 0, 0) of "Vysunutí10"
sketch "Náčrt10" plane through (-35.5, -40.5, 11.95) normal (0, -1, 0) x (1, 0, 0)
  line L0 (101.2872, -38.95) -> (105.5, -23.2276) projected
  line L1 (105.5, -13.95) -> (105.5, -23.2276) projected
  line L2 (107.5, -11.95) -> (105.5, -13.95) projected
  line L3 (107.5, -11.95) -> (149.5, -11.95) projected
  line L4 (149.5, -11.95) -> (149.5, 0) projected
  line L5 (0, 0) -> (149.5, 0) projected
  line L6 (0, -11.95) -> (0, 0) projected
  line L7 (0, -11.95) -> (85.5, -11.95) projected
  line L8 (85.5, -11.95) -> (85.5, -38.95) projected
  line L9 (85.5, -38.95) -> (101.2872, -38.95) projected
  line L10 (89.86, -9.6512) -> (101.14, -9.6512) construction
  line L11 (101.14, -9.6512) -> (101.14, -27.5264) construction
  line L12 (101.14, -27.5264) -> (89.86, -27.5264) construction
  line L13 (89.86, -27.5264) -> (89.86, -9.6512) construction
  line L14 (147.3246, 0) -> (43.6754, 0) projected
  line L15 (96.0421, -21.5815) -> (94.2091, -21.5815)
  line L16 (94.2091, -21.5815) -> (92.5413, -19.3789)
  line L17 (92.5413, -19.3789) -> (91.9968, -19.3789)
  line L18 (91.9968, -19.3789) -> (91.9968, -21.5815)
  line L19 (91.9968, -21.5815) -> (90.4992, -21.5815)
  line L20 (90.4992, -21.5815) -> (90.4992, -15.5815)
  line L21 (90.4992, -15.5815) -> (92.9109, -15.5815)
  spline S0 degree 2 poles (92.9109, -15.5815) (93.4117, -15.5815) (94.1507, -15.7079) (94.4668, -15.9024) knots 0 0 0 1 2 2 2
  spline S1 degree 2 poles (94.4668, -15.9024) (94.7877, -16.1066) (95.1669, -16.7436) (95.1669, -17.2298) knots 0 0 0 1 2 2 2
  spline S2 degree 2 poles (95.1669, -17.2298) (95.1669, -17.9154) (94.5446, -18.776) (94.0243, -19.0288) knots 0 0 0 1 2 2 2
  line L22 (94.0243, -19.0288) -> (96.0421, -21.5815)
  spline S3 degree 2 poles (93.6207, -17.4194) (93.6207, -17.1909) (93.4457, -16.8651) (93.2464, -16.7776) knots 0 0 0 1 2 2 2
  spline S4 degree 2 poles (93.2464, -16.7776) (93.1053, -16.7193) (92.7601, -16.6852) (92.5024, -16.6852) knots 0 0 0 1 2 2 2
  line L23 (92.5024, -16.6852) -> (91.9968, -16.6852)
  line L24 (91.9968, -16.6852) -> (91.9968, -18.2995)
  line L25 (91.9968, -18.2995) -> (92.4295, -18.2995)
  spline S5 degree 2 poles (92.4295, -18.2995) (92.7407, -18.2995) (93.1831, -18.2217) (93.3339, -18.1001) knots 0 0 0 1 2 2 2
  spline S6 degree 2 poles (93.3339, -18.1001) (93.4797, -17.9834) (93.6207, -17.6723) (93.6207, -17.4194) knots 0 0 0 1 2 2 2
  line L26 (100.9579, -20.1812) -> (100.1459, -20.1812)
  line L27 (100.1459, -20.1812) -> (100.1459, -21.5961)
  line L28 (100.1459, -21.5961) -> (98.6921, -21.5961)
  line L29 (98.6921, -21.5961) -> (98.6921, -20.1812)
  line L30 (98.6921, -20.1812) -> (96.047, -20.1812)
  line L31 (96.047, -20.1812) -> (96.047, -19.0629)
  line L32 (96.047, -19.0629) -> (98.6434, -15.5815)
  line L33 (98.6434, -15.5815) -> (100.1459, -15.5815)
  line L34 (100.1459, -15.5815) -> (100.1459, -19.1018)
  line L35 (100.1459, -19.1018) -> (100.9579, -19.1018)
  line L36 (100.9579, -19.1018) -> (100.9579, -20.1812)
  line L37 (98.6921, -19.1018) -> (98.6921, -17.0596)
  line L38 (98.6921, -17.0596) -> (97.1702, -19.1018)
  line L39 (97.1702, -19.1018) -> (98.6921, -19.1018)
  point P0 (35.5, -11.95)
  point P1 (95.5, -27.5264)
  point P2 (95.5, 0)
  point P3 (89.86, -18.5888)
  point P4 (105.5, -18.5888)
  dimension "rev_num" = 4
  constraints: 4 midpoint, 1 horizontal alignment, 1 vertical alignment, 2 other
emboss "Reliéf1" sketch "Náčrt10" operation cut depth 0.75 direction (0, 1, 0) contours L15 L16 L17 L18 L19 L20 L21 S0 S1 S2 L22 | L26 L27 L28 L29 L30 L31 L32 L33 L34 L35 L36
ref_plane "Pracovní rovina5" through (0, 0, 5.975) normal (0, 0, 1) x (1, 0, 0)
sketch "Náčrt11" plane through (0, 0, 5.975) normal (0, 0, 1) x (1, 0, 0)
  circle A0 centre (-9.3, -35.6) radius 2.65 projected
  circle A1 centre (-32.55, -12.35) radius 2.65 projected
  circle A2 centre (110.7, -35.6) radius 2.65 projected
  circle A3 centre (87.45, -12.35) radius 2.65 projected
  line L0 (5, 5) -> (-5, 5) projected
  line L1 (-5, 5) -> (-8.1754, -0.5) projected
  line L2 (-8.1754, -0.5) -> (-35.5, -0.5) projected
  line L3 (-35.5, -0.5) -> (-38, -3) projected
  line L4 (-38, -3) -> (-38, -38) projected
  line L5 (-38, -38) -> (-35.5, -40.5) projected
  line L6 (-35.5, -40.5) -> (114, -40.5) projected
  line L7 (114, -40.5) -> (130, -24.5) projected
  line L8 (130, -24.5) -> (130, -3.6603) projected
  line L9 (130, -3.6603) -> (125, 5) projected
  line L10 (125, 5) -> (115, 5) projected
  line L11 (115, 5) -> (111.8246, -0.5) projected
  line L12 (111.8246, -0.5) -> (8.1754, -0.5) projected
  line L13 (8.1754, -0.5) -> (5, 5) projected
  arc A4 (0.375, -4.0577) -> (-0.375, -4.0577) centre (0, 0) ccw projected
  line L14 (0.375, -12) -> (0.375, -4.0577) projected
  line L15 (-0.375, -12) -> (0.375, -12) projected
  line L16 (-0.375, -4.0577) -> (-0.375, -12) projected
  arc A5 (120.375, -4.0577) -> (119.625, -4.0577) centre (120, 0) ccw projected
  line L17 (120.375, -12) -> (120.375, -4.0577) projected
  line L18 (119.625, -12) -> (120.375, -12) projected
  line L19 (119.625, -4.0577) -> (119.625, -12) projected
  circle A6 centre (-32.55, -12.35) radius 3.6
  circle A7 centre (-9.3, -35.6) radius 3.6
  circle A8 centre (110.7, -35.6) radius 3.6
  circle A9 centre (87.45, -12.35) radius 3.6
  line L20 (-37.15, -3.3521) -> (-35.1479, -1.35)
  line L21 (-35.1479, -1.35) -> (-7.6847, -1.35)
  line L22 (-7.6847, -1.35) -> (-4.5093, 4.15)
  line L23 (-4.5093, 4.15) -> (4.5093, 4.15)
  line L24 (4.5093, 4.15) -> (7.6847, -1.35)
  line L25 (7.6847, -1.35) -> (112.3153, -1.35)
  line L26 (112.3153, -1.35) -> (115.4907, 4.15)
  line L27 (115.4907, 4.15) -> (124.5093, 4.15)
  line L28 (124.5093, 4.15) -> (129.15, -3.888)
  line L29 (129.15, -3.888) -> (129.15, -24.1479)
  line L30 (129.15, -24.1479) -> (113.6479, -39.65)
  line L31 (113.6479, -39.65) -> (-35.1479, -39.65)
  line L32 (-35.1479, -39.65) -> (-37.15, -37.6479)
  line L33 (-37.15, -37.6479) -> (-37.15, -3.3521)
  line L34 (1.225, -4.7702) -> (1.225, -12.85)
  line L35 (1.225, -12.85) -> (-1.225, -12.85)
  line L36 (-1.225, -12.85) -> (-1.225, -4.7702)
  line L37 (118.775, -4.7702) -> (118.775, -12.85)
  line L38 (118.775, -12.85) -> (121.225, -12.85)
  line L39 (121.225, -12.85) -> (121.225, -4.7702)
  arc A10 (121.225, -4.7702) -> (122.652, 4.15) centre (120, 0) ccw
  arc A11 (117.348, 4.15) -> (118.775, -4.7702) centre (120, 0) ccw
  arc A12 (1.225, -4.7702) -> (2.652, 4.15) centre (0, 0) ccw
  arc A13 (-2.652, 4.15) -> (-1.225, -4.7702) centre (0, 0) ccw
  dimension "d197" = 0.95
  dimension "d198" = 0.85
  dimension "d200" = 0.85
  dimension "d201" = 0.85
  dimension "d202" = 0.85
  constraints: 40 end point, 8 centre point, 8 point on circle, 6 equal radius, 4 point on line, 17 other
  measures "d197" radial gap between concentric circles of A6 A1
  measures "d198" distance between parallel lines of L3 L20
  measures "d200" distance between parallel lines of L17 L39
  measures "d201" radial gap between concentric circles of A13 A4
  measures "d202" distance between parallel lines of L36 L16
extrude "Vysunutí11" [suppressed]
sketch "Náčrt12" plane through (0, 0, 11.95) normal (0, 0, 1) x (1, 0, 0)
  circle A0 centre (-9.3, -35.6) radius 2.65 projected
  circle A1 centre (-32.55, -12.35) radius 2.65 projected
  circle A2 centre (110.7, -35.6) radius 2.65 projected
  circle A3 centre (87.45, -12.35) radius 2.65 projected
  line L0 (5, 5) -> (-5, 5) projected
  line L1 (-5, 5) -> (-8.1754, -0.5) projected
  line L2 (-8.1754, -0.5) -> (-35.5, -0.5) projected
  line L3 (-35.5, -0.5) -> (-38, -3) projected
  line L4 (-38, -3) -> (-38, -38) projected
  line L5 (-38, -38) -> (-35.5, -40.5) projected
  line L6 (-35.5, -40.5) -> (114, -40.5) projected
  line L7 (114, -40.5) -> (130, -24.5) projected
  line L8 (130, -24.5) -> (130, -3.6603) projected
  line L9 (130, -3.6603) -> (125, 5) projected
  line L10 (125, 5) -> (115, 5) projected
  line L11 (115, 5) -> (111.8246, -0.5) projected
  line L12 (111.8246, -0.5) -> (8.1754, -0.5) projected
  line L13 (8.1754, -0.5) -> (5, 5) projected
  line L14 (-35.5, -40.5) -> (114, -40.5) projected
  arc A4 (-11.9264, -45.1852) -> (13.0736, -40.5) centre (-13.2553, 30.9483) ccw
  line L15 (-11.9264, -45.1852) -> (-29.9236, -45.4993)
  arc A5 (-11.9686, -42.7655) -> (4.9251, -40.5) centre (-13.2553, 30.9483) ccw
  line L16 (-11.9686, -42.7655) -> (-29.9659, -43.0797)
  arc A6 (-34.1983, -42.6594) -> (-29.9236, -45.4993) centre (-30.0025, -40.9808) ccw
  arc A7 (-31.9515, -41.7606) -> (-34.1983, -42.6594) centre (-33.0749, -42.21) ccw
  arc A8 (-31.9515, -41.7606) -> (-29.9659, -43.0797) centre (-30.0025, -40.9808) ccw
  arc A9 (73.2249, -40.5) -> (90.1186, -42.7655) centre (91.4053, 30.9483) ccw
  line L17 (90.1186, -42.7655) -> (108.1159, -43.0797)
  arc A10 (65.0764, -40.5) -> (90.0764, -45.1852) centre (91.4053, 30.9483) ccw
  line L18 (90.0764, -45.1852) -> (108.0736, -45.4993)
  arc A11 (108.1159, -43.0797) -> (110.1015, -41.7606) centre (108.1525, -40.9808) ccw
  arc A12 (112.3483, -42.6594) -> (110.1015, -41.7606) centre (111.2249, -42.21) ccw
  arc A13 (108.0736, -45.4993) -> (112.3483, -42.6594) centre (108.1525, -40.9808) ccw
  line L19 (65.0764, -40.5) -> (73.2249, -40.5)
  line L20 (4.9251, -40.5) -> (13.0736, -40.5)
  line L21 (-35.5, -40.5) -> (50, -40.5) projected
  line L22 (-71.6, 0) -> (163.6, 0) projected
  line L23 (0, -61.6734) -> (0, 46.3853) projected
  point P0 (0, 0)
  point P1 (-20.925, -45.3422)
  point P2 (99.075, -45.3422)
  point P3 (99.075, -45.3422)
  dimension "d210" = 18
  dimension "d212" = 11.625
  dimension "d213" = 25
  dimension "d214" = 11.625
  dimension "d215" = 2.42
  dimension "d216" = 0.5
  dimension "d217" = 38
  dimension "d220" = 1
  dimension "d222" = 5
  dimension "d223" = 1
  constraints: 20 point on circle, 12 end point, 11 tangent, 10 centre point, 4 equal radius, 4 point on line, 2 collinear, 2 equal length, 2 horizontal alignment, 2 midpoint, 1 coincident, 1 concentric, 1 parallel, 1 other
  measures "d210" distance of L15.start L15.end
  measures "d212" horizontal distance of A1.centre point (-20.925, -45.342)
  measures "d213" horizontal distance of L20.end L15.start
  measures "d214" horizontal distance of A3.centre point (99.075, -45.342)
  measures "d215" radial gap between concentric circles of A4 A5
  measures "d216" distance edge to line of A7 L14
  measures "d217" horizontal distance of L20.start A7.centre
  measures "d220" angle of L6 L16
  measures "d223" angle of L6 L17
extrude "Vysunutí12" [suppressed]
sketch "Náčrt13" plane through (0, 0, 11.95) normal (0, 0, 1) x (1, 0, 0)
  circle A0 centre (-9.3, -35.6) radius 2.65 projected
  circle A1 centre (-32.55, -12.35) radius 2.65 projected
  circle A2 centre (110.7, -35.6) radius 2.65 projected
  circle A3 centre (87.45, -12.35) radius 2.65 projected
  line L0 (5, 5) -> (-5, 5) projected
  line L1 (-5, 5) -> (-8.1754, -0.5) projected
  line L2 (-8.1754, -0.5) -> (-35.5, -0.5) projected
  line L3 (-35.5, -0.5) -> (-38, -3) projected
  line L4 (-38, -3) -> (-38, -38) projected
  line L5 (-38, -38) -> (-35.5, -40.5) projected
  line L6 (-35.5, -40.5) -> (114, -40.5) projected
  line L7 (114, -40.5) -> (130, -24.5) projected
  line L8 (130, -24.5) -> (130, -3.6603) projected
  line L9 (130, -3.6603) -> (125, 5) projected
  line L10 (125, 5) -> (115, 5) projected
  line L11 (115, 5) -> (111.8246, -0.5) projected
  line L12 (111.8246, -0.5) -> (8.1754, -0.5) projected
  line L13 (8.1754, -0.5) -> (5, 5) projected
  line L14 (-25.4, -5.95) -> (21.6, -5.95) construction
  line L15 (21.6, -5.95) -> (21.6, -13.15) construction
  line L16 (21.6, -13.15) -> (-25.4, -13.15) construction
  line L17 (-25.4, -13.15) -> (-25.4, -5.95) construction
  line L18 (-25.4, -18.15) -> (21.6, -18.15) construction
  line L19 (21.6, -18.15) -> (21.6, -27.65) construction
  line L20 (21.6, -27.65) -> (-25.4, -27.65) construction
  line L21 (-25.4, -27.65) -> (-25.4, -18.15) construction
  line L22 (25.6, -5.95) -> (80.6, -5.95) construction
  line L23 (80.6, -5.95) -> (80.6, -27.65) construction
  line L24 (80.6, -27.65) -> (25.6, -27.65) construction
  line L25 (25.6, -27.65) -> (25.6, -5.95) construction
  circle A4 centre (-9.3, -35.6) radius 5
  point P0 (0, 0)
  point P1 (-1.9, -5.95)
  dimension "d224" = 4
  dimension "d225" = 7.2
  dimension "d226" = 9.5
  dimension "d227" = 47
  dimension "d228" = 5
  dimension "d229" = 55
  dimension "d231" = 10
  dimension "d237" = 4.5
  dimension "d238" = 5.45
  constraints: 4 collinear, 1 centre point, 1 horizontal, 1 midpoint, 6 other
  measures "d224" distance between parallel lines of L25 L15
  measures "d225" distance of L16.end L14.start
  measures "d226" distance of L20.end L18.start
  measures "d227" distance between parallel lines of L17 L15
  measures "d228" distance between parallel lines of L18 L16
  measures "d229" distance of L22.start L22.end
  measures "d231" diameter of A4
  measures "d237" distance edge to line of A1 L17
  measures "d238" distance between parallel lines of L2 L14
feature "Reliéf2" [suppressed]
chamfer "Zkosení3" distance 0.5 angle 70 18 edges at (84.8, -12.35, 11.95) (108.05, -35.6, 11.95) (-35.2, -12.35, 11.95) (-11.95, -35.6, 11.95) (-6.5877, 2.25, 11.95) (0, 5, 11.95) (6.5877, 2.25, 11.95) (60, -0.5, 11.95) (-21.8377, -0.5, 11.95) (113.4123, 2.25, 11.95) (120, 5, 11.95) (127.5, 0.6699, 11.95) (130, -14.0801, 11.95) (122, -32.5, 11.95) (39.25, -40.5, 11.95) (-36.75, -39.25, 11.95) (-38, -20.5, 11.95) (-36.75, -1.75, 11.95) measured on face at (6.1547, 2, 11.95) measured on face at (121.6464, -32.1464, 11.95) measured on face at (84.3, -12.35, 11.95) measured on face at (107.55, -35.6, 11.95) measured on face at (-37.5, -20.5, 11.95) measured on face at (60, -1, 11.95) measured on face at (-12.45, -35.6, 11.95) measured on face at (-36.3964, -2.1036, 11.95) measured on face at (-35.7, -12.35, 11.95) measured on face at (-6.1547, 2, 11.95) measured on face at (-36.3964, -38.8964, 11.95) measured on face at (120, 4.5, 11.95) measured on face at (113.8453, 2, 11.95) measured on face at (129.5, -14.0801, 11.95) measured on face at (127.067, 0.4199, 11.95) measured on face at (-21.8377, -1, 11.95) measured on face at (39.25, -40, 11.95) measured on face at (0, 4.5, 11.95)
ref_plane "Pracovní rovina7" through (0, -33.975, 0) normal (0, 1, 0) x (-1, 0, 0)
sketch "Náčrt14" plane through (0, -33.975, 0) normal (0, 1, 0) x (-1, 0, 0)
  line L0 (-113.7929, 11.95) -> (35.2929, 11.95) projected
  line L1 (-129.5, 11.95) -> (-113.7929, 11.95) projected
  line L2 (-124.7113, 11.95) -> (-129.5, 11.95) projected
  line L3 (-115.2887, 11.95) -> (-124.7113, 11.95) projected
  line L4 (-112.1132, 11.95) -> (-115.2887, 11.95) projected
  line L5 (-7.8868, 11.95) -> (-112.1132, 11.95) projected
  line L6 (-4.7113, 11.95) -> (-7.8868, 11.95) projected
  line L7 (4.7113, 11.95) -> (-4.7113, 11.95) projected
  line L8 (7.8868, 11.95) -> (4.7113, 11.95) projected
  line L9 (35.2929, 11.95) -> (7.8868, 11.95) projected
  line L10 (37.5, 11.95) -> (35.2929, 11.95) projected
  line L11 (35.2929, 11.95) -> (37.5, 11.95) projected
  line L12 (35.7, 11.95) -> (29.4, 11.95) projected
  line L13 (-84.3, 11.95) -> (-90.6, 11.95) projected
  line L14 (-107.55, 11.95) -> (-113.85, 11.95) projected
  line L15 (12.45, 11.95) -> (6.15, 11.95) projected
  line L16 (37.5, 11.95) -> (38, 10.5763) projected
  line L17 (37.5, 11.95) -> (38, 10.5763) projected
  line L18 (38, 0) -> (38, 10.5763) projected
  line L19 (38, 0) -> (38, 10.5763) projected
  line L20 (38, 8.45) -> (30, 11.95)
  line L21 (29.9659, 11.95) -> (31.9515, 11.95) projected
  line L22 (38, 0) -> (38, 10.5763) projected
  line L23 (38, 8.45) -> (38, 10.5763)
  line L24 (38, 10.5763) -> (37.5, 11.95)
  line L25 (11.9686, 11.95) -> (29.9659, 11.95) projected
  line L26 (29.9659, 11.95) -> (37.5, 11.95)
  line L27 (30, 11.95) -> (27.8793, 11.95)
  line L28 (27.8793, 11.95) -> (38, 7.5222)
  line L29 (38, 7.5222) -> (38, 8.45)
  line L30 (37.5, 11.95) -> (38, 10.5763) projected
  line L31 (38, 8.45) -> (38, 10.5763)
  line L32 (38, 10.5763) -> (37.5, 11.95)
  line L33 (37.5, 11.95) -> (30, 11.95)
  line L34 (34.1983, 11.95) -> (29.9236, 11.95) projected
  point P0 (0, 0)
  point P1 (15.5742, 11.95)
  point P2 (15.5742, 11.95)
  point P3 (13.6553, 11.95)
  point P4 (13.6553, 11.95)
  point P5 (24.4297, 11.95)
  point P6 (24.4297, 11.95)
  point P7 (21.3524, 11.95)
  point P8 (19.0715, 11.95)
  point P9 (17.1527, 11.95)
  point P10 (19.2742, 11.95)
  point P11 (21.2582, 11.95)
  point P12 (22.5109, 11.95)
  point P13 (22.5109, 11.95)
  point P14 (13.1457, 11.95)
  point P15 (15.0884, 11.95)
  point P16 (15.3848, 11.95)
  point P17 (15.3848, 11.95)
  point P18 (16.839, 11.95)
  point P19 (16.839, 11.95)
  point P20 (13.7768, 11.95)
  point P21 (21.4762, 11.95)
  point P22 (17.975, 11.95)
  point P23 (21.4598, 11.95)
  point P24 (24.961, 11.95)
  point P25 (24.6317, 11.95)
  point P26 (23.0293, 11.95)
  dimension "d243" = 8
  dimension "d244" = 3.5
  dimension "d247" = 0.85
  constraints: 20 end point, 6 collinear, 3 point on line, 1 parallel, 1 vertical, 2 other
  measures "d243" horizontal distance of L20.start L20.end
  measures "d244" vertical distance of L20.start L20.end
  measures "d247" distance between parallel lines of L20 L28
extrude "Vysunutí14" cut sketch "Náčrt14" along normal blind 11.5
extrude "Vysunutí15" add sketch "Náčrt14" along normal blind 11.5 contours L0 L20 L18 L28
move faces "Otočit1" rotation origin (0, 0, 0) rotation axis (1, 0, 0) rotation angle 20 translate (0, 0.8411, 12.1297) faces at (-35.3333, -33.975, 10.3254)
move faces "Otočit2" rotation origin (0, 0, 0) rotation axis (1, 0, 0) rotation angle -20 translate (0, -4.2455, -7.1773) faces at (-35.3333, -22.475, 10.3254)
chamfer "Zkosení4" distance 0.4 angle 70 1 edges at (120, 4.075, 0) measured on face at (120, 4.575, 0)